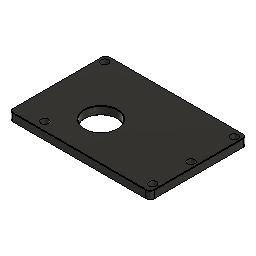
ServoPlate (Autodesk Fusion 360 design; units mm, degrees)
Autodesk Fusion 360 part; units mm, degrees
note: some values were not read from the file. Chosen so that the rebuilt part matches the saved one: which face or edge a step refers to. Set by a fixed rule: which sketch regions a step uses.
sketch "Sketch1" plane through (0, 0, 0) normal (0, 0, 1) x (1, 0, 0)
  circle A0 centre (18.7728, 42.4051) radius 2.159
  line L0 (-60.9197, 30.0451) -> (-60.9197, 69.4151)
  line L1 (22.2603, 30.0451) -> (22.2603, 69.4151)
  line L2 (19.7203, 71.9551) -> (-58.3797, 71.9551)
  arc A1 (-58.3797, 71.9551) -> (-60.9197, 69.4151) centre (-58.3797, 69.4151) ccw
  arc A2 (22.2603, 69.4151) -> (19.7203, 71.9551) centre (19.7203, 69.4151) ccw
  line L3 (-60.9197, 71.9551) -> (22.2603, 71.9551)
  circle A3 centre (-57.4272, 67.8053) radius 2.159
  circle A4 centre (18.7728, 67.8053) radius 2.159
  circle A5 centre (-44.7272, 19.9053) radius 2.159
  circle A6 centre (18.7728, 19.9051) radius 2.159
  line L4 (-60.9197, 30.0451) -> (-60.9197, 17.3451)
  line L5 (22.2603, 30.0451) -> (22.2603, 17.3451)
  line L6 (19.7203, 14.8051) -> (3.2103, 14.8051)
  line L7 (-41.8697, 14.8051) -> (-58.3797, 14.8051)
  arc A7 (-60.9197, 17.3451) -> (-58.3797, 14.8051) centre (-58.3797, 17.3451) ccw
  arc A8 (19.7203, 14.8051) -> (22.2603, 17.3451) centre (19.7203, 17.3451) ccw
  line L8 (-41.8697, 14.8051) -> (3.2103, 14.8051)
  line L9 (-60.9197, 34.7366) -> (-29.1697, 34.7366)
  line L10 (-28.759, 14.8051) -> (-28.759, 38.3051)
  circle A9 centre (-30.3427, 38.3051) radius 9.5885
  arc A10 (-57.0819, 34.7366) -> (-57.7726, 34.7366) centre (-57.4272, 32.6053) ccw
  point P0 (-54.3297, 57.5051)
  point P1 (-60.9197, 27.5051)
  point P2 (-60.9197, 71.9551)
  point P3 (22.2603, 27.5051)
  point P4 (22.2603, 71.9551)
  point P5 (-60.9197, 14.8051)
  point P6 (22.2603, 14.8051)
  dimension "d37" = 4.318
  dimension "d42" = 4.318
  dimension "d49" = 44.45
  dimension "d51" = 44.45
  dimension "d52" = 2.54
  dimension "d54" = 4.318
  dimension "d66" = 4.318
  dimension "d84" = 4.318
  dimension "d86" = 4.318
  dimension "d89" = 15.24
  dimension "d90" = 15.24
  dimension "d93" = 2.54
  dimension "d106" = 31.75
  dimension "d107" = 23.5
  dimension "d108" = 19.177
  constraint coincident P2 L0
  constraint coincident P2 L2
  constraint tangent L0 A1
  constraint tangent L2 A1
  constraint coincident P4 L1
  constraint coincident P4 L2
  constraint tangent L1 A2
  constraint tangent L2 A2
  constraint equal A1 A2
  constraint coincident P3 L1
  constraint coincident P1 L0
  constraint coincident P2 L3.start
  constraint coincident P4 L3.end
  constraint collinear L6 L7
  constraint coincident P5 L4
  constraint coincident P5 L7
  constraint tangent L4 A7
  constraint tangent L7 A7
  constraint coincident P6 L5
  constraint coincident P6 L6
  constraint tangent L5 A8
  constraint tangent L6 A8
  constraint equal A7 A8
  constraint coincident L0 L9.start
  constraint perpendicular L0 L9
  constraint coincident L8 L10.start
  constraint perpendicular L8 L10
  constraint coincident L9 A10.end
  constraint coincident L9 A10.start
  measures "d37" diameter of A0
  measures "d42" diameter of A10
  measures "d49" distance of P1 P2
  measures "d51" distance of P3 P4
  measures "d52" radius of A1
  measures "d54" diameter of A3
  measures "d66" diameter of A4
  measures "d84" diameter of A5
  measures "d86" diameter of A6
  measures "d89" distance of L0.start P5
  measures "d90" distance of L1.start P6
  measures "d93" radius of A7
  measures "d106" distance of L9.start L9.end
  measures "d107" distance of L10.start L10.end
  measures "d108" diameter of A9
extrude "Extrude4" add sketch "Sketch1" along normal blind 4.7625
fillet "Fillet5" radius 0.254 28 edges at (-60.9197, 32.3908, 0) (-60.9197, 32.3908, 4.7625) (-60.9197, 23.6951, 0) (-60.9197, 23.6951, 4.7625) (-60.1758, 15.549, 0) (-60.1758, 15.549, 4.7625) (-50.1247, 14.8051, 0) (-50.1247, 14.8051, 4.7625) (-35.3144, 14.8051, 0) (-35.3144, 14.8051, 4.7625) (-12.7744, 14.8051, 0) (-12.7744, 14.8051, 4.7625) (11.4653, 14.8051, 0) (11.4653, 14.8051, 4.7625) (21.5163, 15.549, 0) (21.5163, 15.549, 4.7625) (22.2603, 23.6951, 0) (22.2603, 23.6951, 4.7625) (22.2603, 49.7301, 0) (22.2603, 49.7301, 4.7625) (21.5163, 71.2111, 0) (21.5163, 71.2111, 4.7625) (-19.3297, 71.9551, 0) (-19.3297, 71.9551, 4.7625) (-60.1758, 71.2111, 0) (-60.1758, 71.2111, 4.7625) (-60.9197, 52.0758, 0) (-60.9197, 52.0758, 4.7625)
sketch "Sketch4" plane through (0, 0, 4.7625) normal (0, 0, 1) x (-1, 0, 0)
  circle A0 centre (44.7272, -19.9053) radius 2.159
  circle A1 centre (-18.7728, -42.4051) radius 2.159
  circle A2 centre (-18.7728, -67.8053) radius 2.159
  circle A3 centre (57.4272, -67.8053) radius 2.159
  circle A4 centre (-18.7728, -19.9051) radius 2.159
  line L0 (58.3797, -15.0591) -> (-19.7203, -15.0591)
  arc A5 (-19.7203, -15.0591) -> (-22.0063, -17.3451) centre (-19.7203, -17.3451) ccw
  line L1 (-22.0063, -17.3451) -> (-22.0063, -69.4151)
  arc A6 (-22.0063, -69.4151) -> (-19.7203, -71.7011) centre (-19.7203, -69.4151) ccw
  line L2 (-19.7203, -71.7011) -> (58.3797, -71.7011)
  arc A7 (58.3797, -71.7011) -> (60.6657, -69.4151) centre (58.3797, -69.4151) ccw
  line L3 (60.6657, -69.4151) -> (60.6657, -17.3451)
  arc A8 (60.6657, -17.3451) -> (58.3797, -15.0591) centre (58.3797, -17.3451) ccw
  line L4 (29.4237, -15.0591) -> (29.4237, -37.5591)
  circle A9 centre (29.4237, -37.5591) radius 9.5885
  line L5 (60.6657, -37.5591) -> (29.4237, -37.5591)
  dimension "d110" = 22.5
  dimension "d111" = 19.177
  dimension "d139" = 31.242
  constraint coincident L0 L4.start
  constraint perpendicular L0 L4
  constraint coincident L4.end A9.centre
  constraint coincident L3 L5.start
  constraint perpendicular L4 L5
  measures "d110" distance of L4.start L4.end
  measures "d111" diameter of A9
  measures "d139" distance of L5.start L4.end
extrude "Extrude6" cut sketch "Sketch4" against normal up to surface (4.7625 mm away) contours L4 A9 L5 | L4 A9 L5
fillet "Fillet7" radius 0.254 2 edges at (-20.4841, 41.0264, 0) (-20.4841, 34.0917, 4.7625)
sketch "Sketch5" plane through (0, 0, 4.7625) normal (0, 0, 1) x (-1, 0, 0)
  line L0 (58.3797, -15.0591) -> (-19.7203, -15.0591)
  arc A0 (-19.7203, -15.0591) -> (-22.0063, -17.3451) centre (-19.7203, -17.3451) ccw
  line L1 (-22.0063, -17.3451) -> (-22.0063, -69.4151)
  arc A1 (-22.0063, -69.4151) -> (-19.7203, -71.7011) centre (-19.7203, -69.4151) ccw
  line L2 (-19.7203, -71.7011) -> (58.3797, -71.7011)
  arc A2 (58.3797, -71.7011) -> (60.6657, -69.4151) centre (58.3797, -69.4151) ccw
  line L3 (60.6657, -69.4151) -> (60.6657, -17.3451)
  arc A3 (60.6657, -17.3451) -> (58.3797, -15.0591) centre (58.3797, -17.3451) ccw
  circle A4 centre (-18.7728, -19.9051) radius 2.159
  circle A5 centre (57.4272, -67.8053) radius 2.159
  circle A6 centre (-18.7728, -67.8053) radius 2.159
  circle A7 centre (-18.7728, -42.4051) radius 2.159
  circle A8 centre (44.7272, -19.9053) radius 2.159
  circle A9 centre (29.4237, -37.5591) radius 9.8425
  line L4 (-18.7728, -42.4051) -> (-18.7728, -48.7551)
  line L5 (-22.0063, -48.7551) -> (-16.9198, -48.7551)
  line L6 (-18.7728, -32.6051) -> (-18.7728, -26.2551)
  line L7 (-14.3798, -46.2151) -> (-14.3798, -28.7904)
  line L8 (-16.9198, -26.2504) -> (-22.0063, -26.2504)
  arc A10 (-16.9198, -48.7551) -> (-14.3798, -46.2151) centre (-16.9198, -46.2151) ccw
  line L9 (-22.0063, -48.7551) -> (-22.2606, -48.7551)
  line L10 (-22.0063, -26.2504) -> (-22.2606, -26.2504)
  arc A11 (-14.3798, -28.7904) -> (-16.9198, -26.2504) centre (-16.9198, -28.7904) ccw
  line L11 (-22.2606, -48.7551) -> (-22.2606, -26.2504)
  dimension "d116" = 6.35
  dimension "d117" = 6.35
  dimension "d118" = 2.54
  dimension "d119" = 2.54
  constraint coincident A7.centre L4.start
  constraint parallel L1 L4
  constraint coincident L1 L5.start
  constraint perpendicular L4 L5
  constraint parallel L1 L6
  constraint perpendicular L5 L7
  constraint coincident L1 L8.end
  constraint perpendicular L1 L8
  constraint tangent L5 A10
  constraint tangent L7 A10
  constraint perpendicular L1 L9
  constraint perpendicular L1 L10
  constraint tangent L7 A11
  constraint tangent L8 A11
  constraint perpendicular L10 L11
  measures "d116" distance of A7.centre L4.end
  measures "d117" distance of L6.start L6.end
  measures "d118" radius of A10
  measures "d119" radius of A11
sketch "Sketch6" plane through (22.2606, 0, 0) normal (1, 0, 0) x (0, 1, 0)
  line L0 (26.2504, 4.7625) -> (48.7551, 4.7625)
  line L1 (48.7551, 4.7625) -> (48.7551, 9.525)
  line L2 (48.7551, 9.525) -> (26.2504, 9.525)
  line L3 (26.2504, 9.525) -> (26.2504, 4.7625)
sketch "Sketch7" plane through (22.2606, 0, 0) normal (1, 0, 0) x (0, 1, 0)
  line L0 (26.2504, 9.5249) -> (48.7567, 9.5249)
  line L1 (48.7567, 9.5249) -> (48.7567, -52)
  line L2 (48.7567, -52) -> (26.2504, -52)
  line L3 (26.2504, -52) -> (26.2504, 9.5249)
  dimension "d122" = 61.5249
  constraint horizontal L0
  constraint vertical L1
  constraint horizontal L2
  constraint vertical L3
  measures "d122" distance of L0.start L2.end
sketch "Sketch8" plane through (0, 0, -52) normal (0, 0, -1) x (1, 0, 0)
  line L0 (22.2606, -26.2504) -> (22.2606, -48.7567)
  line L1 (22.2606, -48.7567) -> (27.0231, -48.7567)
  line L2 (27.0231, -48.7567) -> (27.0231, -26.2504)
  line L3 (27.0231, -26.2504) -> (22.2606, -26.2504)
  line L4 (22.2606, -26.2504) -> (17.1806, -26.2504)
  line L5 (22.2606, -48.7567) -> (17.1806, -48.7567)
  line L6 (14.6406, -46.2167) -> (14.6406, -28.7904)
  arc A0 (17.1806, -26.2504) -> (14.6406, -28.7904) centre (17.1806, -28.7904) ccw
  arc A1 (14.6406, -46.2167) -> (17.1806, -48.7567) centre (17.1806, -46.2167) ccw
  line L7 (18.7728, -48.7551) -> (18.7728, -26.2504)
  circle A2 centre (18.7728, -42.4051) radius 2.159
  circle A3 centre (18.7728, -32.6051) radius 2.159
  point P0 (14.6406, -26.2504)
  point P1 (14.6406, -48.7567)
  dimension "d125" = 7.62
  dimension "d126" = 7.62
  dimension "d127" = 2.54
  dimension "d128" = 4.318
  dimension "d129" = 4.318
  constraint coincident L0.start L3.end
  constraint perpendicular L0 L4
  constraint coincident L0.end L1.start
  constraint perpendicular L0 L5
  constraint coincident P0 L4
  constraint coincident P0 L6
  constraint tangent L4 A0
  constraint tangent L6 A0
  constraint coincident P1 L5
  constraint coincident P1 L6
  constraint tangent L5 A1
  constraint tangent L6 A1
  constraint equal A0 A1
  constraint coincident L4 L7.end
  constraint perpendicular L4 L7
  constraint coincident L7 A2.centre
  constraint coincident L7 A3.centre
  measures "d125" distance of L0.start P0
  measures "d126" distance of L0.end P1
  measures "d127" radius of A0
  measures "d128" diameter of A2
  measures "d129" diameter of A3
sketch "Sketch9" plane through (27.0231, 0, 0) normal (1, 0, 0) x (0, 1, 0)
  line L0 (26.2504, -52) -> (48.7567, -52)
  line L1 (48.7567, -52) -> (48.7567, 9.5249)
  line L2 (48.7567, 9.5249) -> (26.2504, 9.5249)
  line L3 (26.2504, 9.5249) -> (26.2504, -52)
  line L4 (26.2504, -21.2375) -> (48.7567, -21.2375)
  line L5 (37.5036, -52) -> (37.5036, 9.5249)
  line L6 (37.5036, 9.5249) -> (37.5036, -15.8751)
  line L7 (37.5036, -15.8751) -> (27.5036, -15.8751)
  line L8 (37.5036, -15.8751) -> (47.5036, -15.8751)
  circle A0 centre (42.5036, -15.8751) radius 2.5
  circle A1 centre (32.5036, -15.8751) radius 2.5
  dimension "d132" = 25.4
  dimension "d133" = 10
  dimension "d134" = 10
  dimension "d135" = 5
  dimension "d136" = 5
  constraint midpoint L3 L4.start
  constraint midpoint L1 L4.end
  constraint midpoint L0 L5.start
  constraint midpoint L2 L5.end
  constraint coincident L5 L6.end
  constraint perpendicular L5 L7
  constraint perpendicular L1 L8
  constraint midpoint L8 A0.centre
  constraint midpoint L7 A1.centre
  measures "d132" distance of L5.end L6.end
  measures "d133" distance of L6.end L7.end
  measures "d134" distance of L6.end L8.end
  measures "d135" diameter of A0
  measures "d136" diameter of A1
equation "d94 = ( 3 / 16 ) * 1 in"
equation "d122 = 2.04724 in + 0.375 in"
equation "d134 = cm"
named bodies: "ServoPlate"
